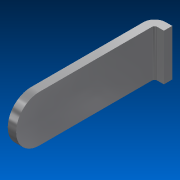
# Autodesk Inventor part: Terminal 3
Saved by Autodesk Inventor 2013 (Build 170138000, 138)
## iProperties
Created: 2012-05-07
Material: Brass, Soft Yellow
Document SubType Name: Modeling
Designer: sdarley
Density: 1 g/cm^3
Project: 2.1mm DC Power Socket
Description: Terminal 3
Author: sdarley
Title: Terminal 3
Revision Number: 1
Autodesk Inventor part; units mm, degrees
ref_plane "YZ Plane" through (0, 0, 0) normal (1, 0, 0) x (0, 1, 0)
ref_plane "XZ Plane" through (0, 0, 0) normal (0, 1, 0) x (-1, 0, 0)
ref_plane "XY Plane" through (0, 0, 0) normal (0, 0, 1) x (1, 0, 0)
sketch "Sketch1" plane through (0, 0, 0) normal (0, 0, 1) x (1, 0, 0)
  line L0 (0, 0) -> (0, -0.45)
  line L1 (0, -0.45) -> (-0.35, -0.45)
  line L2 (0, 0) -> (-0.35, 0)
  arc A0 (-0.35, -0.45) -> (-0.5, -0.6) centre (-0.35, -0.6) ccw
  arc A1 (-0.35, 0) -> (-0.95, -0.6) centre (-0.35, -0.6) ccw
  line L3 (-0.95, -0.6) -> (-0.95, -7.9)
  line L4 (-0.95, -7.9) -> (-0.5, -7.9)
  line L5 (-0.5, -7.9) -> (-0.5, -0.6)
  dimension "d0" = 0.45
  dimension "d2" = 7.9
  dimension "d3" = 0.95
  dimension "d4" = 0.6
  constraints: 12 end point, 4 point on circle, 3 perpendicular, 3 tangent, 2 centre point, 2 parallel, 1 concentric, 1 horizontal alignment, 1 vertical
  measures "d0" distance between parallel lines of L2 L1
  measures "d2" distance between parallel lines of L4 L2
  measures "d3" distance between parallel lines of L0 L3
  measures "d4" vertical distance of L2.end L5.end
extrude "Extrusion1" add sketch "Sketch1" along normal blind 2.5
fillet "Fillet1" radius 1.25 2 edges at (-0.725, -7.9, 2.5) (-0.725, -7.9, 0)
body "Solid1"
